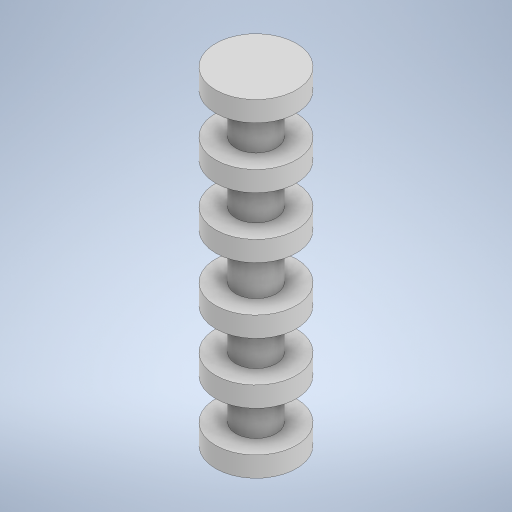
# Autodesk Inventor part: Crankshaft Crank Cylinder
Saved by Autodesk Inventor 2023 (Build 270158000, 158)
## iProperties
Created: 2022-10-29
Part Number: Crankshaft Crank Cylinder
Material: Generic
Document SubType Name: Modeling
Designer: tommy
Density: 1 g/cm^3
Appearance: Default
Author: tommy
Autodesk Inventor part; units mm, degrees
ref_plane "YZ Plane" through (0, 0, 0) normal (1, 0, 0) x (0, 1, 0)
ref_plane "XZ Plane" through (0, 0, 0) normal (0, 1, 0) x (-1, 0, 0)
ref_plane "XY Plane" through (0, 0, 0) normal (0, 0, 1) x (1, 0, 0)
sketch "Sketch1" plane through (0, 0, 0) normal (1, 0, 0) x (0, 1, 0)
  line L0 (0, 0) -> (0, -3.9878)
  line L1 (0, -3.9878) -> (0, -6.35)
  line L2 (0, -6.35) -> (3.175, -6.35)
  line L3 (3.175, -6.35) -> (3.175, -3.175)
  line L4 (3.175, -3.175) -> (9.525, -3.175)
  line L5 (9.525, -3.175) -> (9.525, -6.35)
  line L6 (9.525, -6.35) -> (12.7, -6.35)
  line L7 (12.7, -6.35) -> (12.7, -3.175)
  line L8 (12.7, -3.175) -> (19.05, -3.175)
  line L9 (19.05, -3.175) -> (19.05, -6.35)
  line L10 (19.05, -6.35) -> (22.225, -6.35)
  line L11 (22.225, -6.35) -> (22.225, -3.175)
  line L12 (22.225, -3.175) -> (25.7937, -3.175)
  line L13 (25.7937, 0) -> (0, 0)
  line L14 (51.5874, 0) -> (51.5874, -3.175)
  line L15 (51.5874, -3.175) -> (51.5874, -6.35)
  line L16 (51.5874, -6.35) -> (48.4124, -6.35)
  line L17 (48.4124, -6.35) -> (48.4124, -3.175)
  line L18 (48.4124, -3.175) -> (42.0624, -3.175)
  line L19 (42.0624, -3.175) -> (42.0624, -6.35)
  line L20 (42.0624, -6.35) -> (38.8874, -6.35)
  line L21 (38.8874, -6.35) -> (38.8874, -3.175)
  line L22 (38.8874, -3.175) -> (32.5374, -3.175)
  line L23 (32.5374, -3.175) -> (32.5374, -6.35)
  line L24 (32.5374, -6.35) -> (29.3624, -6.35)
  line L25 (29.3624, -6.35) -> (29.3624, -3.175)
  line L26 (29.3624, -3.175) -> (25.7937, -3.175)
  line L27 (25.7937, 0) -> (51.5874, 0)
  dimension "d1" = 3.9878
  dimension "d2" = 2.3622
  dimension "d3" = 3.175
  dimension "d4" = 6.35
  dimension "d5" = 3.175
  dimension "d6" = 6.35
  dimension "d7" = 3.175
  dimension "d8" = 3.5687
  constraints: 56 end point, 16 point on line, 7 perpendicular, 1 horizontal, 1 vertical
  measures "d1" distance of L0.start L0.end
  measures "d2" distance of L0.end L1.end
  measures "d3" distance of L1.end L2.end
  measures "d4" distance of L3.end L4.end
  measures "d5" distance of L5.end L6.end
  measures "d6" distance of L7.end L8.end
  measures "d7" distance of L9.end L10.end
  measures "d8" distance of L11.end L12.end
revolve "Revolution1" add sketch "Sketch1" angle 360 about axis through (0, 25.7937, 0) along (0, 1, 0)
body "Solid1"
